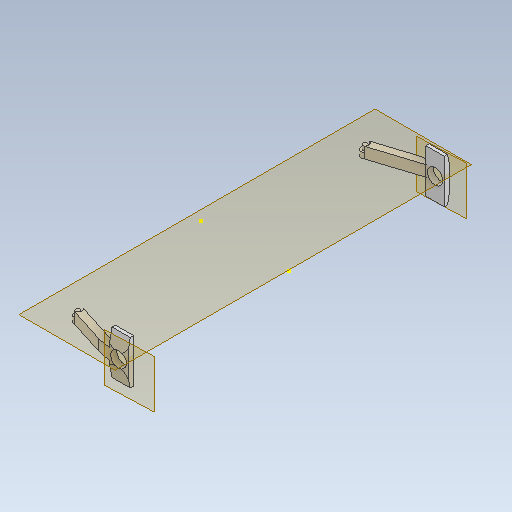
# Autodesk Inventor part: Bauteil16
Saved by Autodesk Inventor 2021 (Build 250183000, 183)
## iProperties
Created: 2021-01-14
Part Number: Bauteil16
Material: Generisch
Document SubType Name: Modeling
Designer: LETPJG
Density: 1 g/cm^3
Appearance: Vorgabe
Author: LETPJG
Autodesk Inventor part; units mm, degrees
ref_plane "YZ Plane" through (0, 0, 0) normal (1, 0, 0) x (0, 1, 0)
ref_plane "XZ Plane" through (0, 0, 0) normal (0, 1, 0) x (-1, 0, 0)
ref_plane "XY Plane" through (0, 0, 0) normal (0, 0, 1) x (1, 0, 0)
sketch "Skizze1" plane through (0, 0, 0) normal (0, 0, 1) x (1, 0, 0)
  point P0 (0, 0)
sketch "Skizze2" plane through (0, 0, 0) normal (0, 1, 0) x (-1, 0, 0)
  line L0 (2.5, 30.2385) -> (-2.5, 30.2385)
  line L1 (-2.5, 30.2385) -> (-2.5, -30.2385)
  line L2 (-2.5, -30.2385) -> (2.5, -30.2385)
  line L3 (2.5, -30.2385) -> (2.5, 30.2385)
  line L4 (-2.5, 49) -> (-2.5, -49)
  line L5 (2.5, -49) -> (2.5, 49)
  circle A0 centre (0, 49) radius 2.5
  circle A1 centre (0, -49) radius 2.5
  line L6 (-9.3293, 67.423) -> (-30, 74)
  line L7 (-7.3602, 65.7604) -> (0, 51.5)
  line L8 (-31.665, 71) -> (-10.3492, 64.2177)
  line L9 (-10.3492, 64.2177) -> (-2.4949, 49)
  line L10 (-31.665, 71) -> (-40, 71)
  line L11 (-30, 74) -> (-40, 74)
  line L12 (-10.3492, 64.2177) -> (-8, 67)
  circle A2 centre (-9.1746, 65.6088) radius 1.8207
  line L13 (-40, 71) -> (-40, 74)
  circle A3 centre (-9.1746, 65.6088) radius 0.9616
  line L14 (-7.3602, -65.7604) -> (0, -51.5)
  circle A4 centre (-9.1746, -65.6088) radius 0.9616
  circle A5 centre (-9.1746, -65.6088) radius 1.8207
  line L15 (-10.3492, -64.2177) -> (-2.4949, -49)
  line L16 (-31.665, -71) -> (-10.3492, -64.2177)
  line L17 (-9.3293, -67.423) -> (-30, -74)
  line L18 (-30, -74) -> (-40, -74)
  line L19 (-40, -71) -> (-40, -74)
  line L20 (-31.665, -71) -> (-40, -71)
  point P0 (0, 0)
  point P1 (0, 0)
  point P2 (0, -30.2385)
  point P3 (2.5, 0)
  point P4 (2.5, 0)
  point P5 (-48.2893, 0)
  dimension "d0" = 5
  constraints: 42 end point, 8 point on circle, 5 centre point, 4 parallel, 3 coincident, 3 horizontal alignment, 3 midpoint, 2 horizontal, 2 vertical alignment, 1 perpendicular, 1 vertical, 2 other
  measures "d0" distance of L1.end L2.end
extrude "Extrusion1" add sketch "Skizze2" along normal mid plane 5 contours L8 L10 L13 L11 L6 A2 | A5 L17 L18 L19 L20 L16
extrude "Extrusion2" add sketch "Skizze2" against normal blind 2.5 contours A2 L12 A3 | A2 L12 A3 | A5 | A3 L12 | L12 A3 | A4
ref_plane "Arbeitsebene1" through (10.3492, 2.5, -64.2177) normal (0, 1, 0) x (1, 0, 0)
sketch "Skizze3" plane through (0, 0, 0) normal (0, 1, 0) x (-1, 0, 0)
  line L0 (-30, 74) -> (-40, 74) projected
  line L1 (-31.665, 71) -> (-10.3492, 64.2177) projected
  line L2 (-40, 74) -> (-31.665, 74)
  line L3 (-31.665, 74) -> (-31.665, 71)
  line L4 (-31.665, 71) -> (-40, 71)
  line L5 (-40, 71) -> (-40, 74)
  line L6 (-40, -71) -> (-40, -74) projected
  line L7 (-31.665, -71) -> (-40, -71) projected
  line L8 (-40, -74) -> (-31.665, -74)
  line L9 (-31.665, -74) -> (-31.665, -71)
  line L10 (-31.665, -71) -> (-40, -71)
  line L11 (-40, -71) -> (-40, -74)
  point P0 (0, 0)
  constraints: 16 end point, 4 parallel, 2 horizontal, 2 perpendicular
extrude "Extrusion3" add sketch "Skizze3" along normal mid plane 20
sketch "Skizze4" plane through (30, -2.5, 74) normal (0, 0, 1) x (1, 0, 0)
  circle A0 centre (5.8325, 2.4963) radius 3.5
  point P0 (-30, 2.5)
  point P1 (1.665, 5)
  dimension "d27" = 7
  constraints: 1 centre point
  measures "d27" diameter of A0
extrude "Extrusion4" cut sketch "Skizze4" against normal blind 150
sketch "Skizze5" plane through (40, -10, 71) normal (1, 0, 0) x (0, 0, -1)
  line L0 (0, 0) -> (0, 7.5) projected
  line L1 (-3, 0) -> (-3, 20) projected
  line L2 (-1.5, 0) -> (-3, 0)
  line L3 (-3, 0) -> (-3, 7.3019)
  line L4 (-3, 12.5) -> (-3, 20) projected
  line L5 (0, 0) -> (0, 20) projected
  line L6 (-3, 20) -> (-1.5, 20)
  line L7 (0, 12.5139) -> (-3, 12.5139)
  line L8 (-3, 12.5139) -> (-3, 20)
  line L9 (0, 20) -> (-3, 20) projected
  line L10 (-1.5, 20) -> (-3, 12.5139)
  line L11 (-3, 0) -> (0, 0) projected
  line L12 (-1.5, 0) -> (-3, 7.3019)
  point P0 (71, 10)
  constraints: 14 end point, 2 horizontal, 2 midpoint, 2 point on line, 1 parallel, 1 perpendicular
extrude "Extrusion5" cut sketch "Skizze5" against normal blind 10 contours L2 L1 L12 | L1 L6 L10
sketch "Skizze6" plane through (40, -10, -74) normal (1, 0, 0) x (0, 0, -1)
  line L0 (-3, 7.5) -> (-3, 0) projected
  line L1 (-3, 0) -> (0, 0) projected
  line L2 (0, 7.5) -> (0, 0)
  line L3 (0, 0) -> (-1.5, 0)
  line L4 (-3, 12.5) -> (0, 12.5) projected
  line L5 (0, 12.5) -> (0, 20) projected
  line L6 (0, 12.5) -> (0, 20)
  line L7 (0, 20) -> (-1.5, 20)
  line L8 (0, 20) -> (-3, 20) projected
  line L9 (-1.5, 20) -> (0, 12.5)
  line L10 (0, 0) -> (0, 7.5) projected
  line L11 (-1.5, 0) -> (0, 7.5)
  point P0 (-74, 10)
  constraints: 12 end point, 1 midpoint
extrude "Extrusion6" cut sketch "Skizze6" against normal blind 10
sketch "Skizze7" plane through (40, -10, -71) normal (1, 0, 0) x (0, 0, -1)
  point P0 (-71, 10)
sketch "Skizze8" plane through (0, -10, 0) normal (0, -1, 0) x (1, 0, 0)
  line L0 (9.3293, -67.423) -> (30, -74) projected
  line L1 (40, -71) -> (40, -72.5) projected
  line L2 (31.665, -74) -> (40, -74) projected
  line L3 (35.8325, -74) -> (40, -74)
  line L4 (40, -74) -> (40, -73.25)
  line L5 (40, -74) -> (40, -72.5) projected
  arc A0 (35.8325, -74) -> (40, -73.25) centre (35.8325, -62.0462) ccw
  line L6 (39.3325, -74) -> (32.3325, -74) projected
  line L7 (40, -72.5) -> (31.665, -72.5) projected
  line L8 (41.6903, 0) -> (29.392, 0)
  line L9 (31.665, 74) -> (40, 74)
  line L10 (40, 74) -> (40, 73.25)
  arc A1 (40, 73.25) -> (35.8325, 74) centre (35.8325, 62.0462) ccw
  point P0 (0, 0)
  point P1 (35.8325, 74)
  constraints: 10 end point, 6 symmetric about line, 4 point on circle, 2 centre point, 2 midpoint, 1 horizontal, 1 tangent, 1 other
extrude "Extrusion7" cut sketch "Skizze8" against normal blind 20
sketch "Skizze9" plane through (0, -10, 0) normal (0, -1, 0) x (1, 0, 0)
  line L0 (31.665, 74) -> (33.5986, 74) projected
  line L1 (40, 72.5) -> (31.665, 72.5) projected
  line L2 (31.665, 74) -> (30, 74) projected
  line L3 (30, 74) -> (35.8325, 74)
  line L4 (9.3293, 67.423) -> (30, 74) projected
  line L5 (30, 74) -> (25.2857, 74)
  line L6 (25.2857, 74) -> (25.2857, 72.5)
  arc A0 (35.8325, 74) -> (25.2857, 72.5) centre (37.5594, 24.0298) ccw
  line L7 (42.1638, 0) -> (18.6987, 0) construction
  line L8 (31.665, -74) -> (35.8325, -74)
  line L9 (31.665, -74) -> (30, -74)
  line L10 (30, -74) -> (25.2857, -74)
  line L11 (25.2857, -74) -> (25.2857, -72.5)
  arc A1 (25.2857, -72.5) -> (35.8325, -74) centre (37.5594, -24.0298) ccw
  point P0 (0, 0)
  point P1 (35.8325, 74)
  point P2 (35.8325, -74)
  point P3 (35.8325, 74)
  constraints: 16 end point, 7 symmetric about line, 4 point on circle, 2 centre point, 2 horizontal, 1 perpendicular, 1 point on line, 1 other
extrude "Extrusion8" cut sketch "Skizze9" against normal blind 20
sketch "Skizze10" plane through (0, 0, 0) normal (0, 1, 0) x (1, 0, 0)
  arc A0 (9.3293, 67.423) -> (10.3492, 64.2177) centre (9.1746, 65.6088) ccw projected
  circle A1 centre (9.1746, 65.6088) radius 1
  line L0 (3.0459, 0) -> (11.7112, 0) construction
  circle A2 centre (9.1746, -65.6088) radius 1
  point P0 (0, 0)
  dimension "d21" = 2
  constraints: 2 centre point, 2 end point, 1 horizontal, 1 symmetric about line, 1 other
  measures "d21" diameter of A1
extrude "Extrusion10" add sketch "Skizze10" along normal blind 2
ref_plane "Arbeitsebene3" through (40.9441, -2.0037, 73.9117) normal (0.0345377, 0, 0.9994034) x (0, 1, 0)
ref_plane "Arbeitsebene2" through (35.8325, -2.0037, -74) normal (0.0345377, 0, 0.9994034) x (0, 1, 0)
